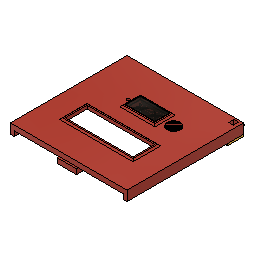
MKTNE_RPI_Shield 3d Files (Autodesk Fusion 360 design; units mm, degrees)
Autodesk Fusion 360 part; units mm, degrees
(part 1 of 2)
sketch "Locking Plug" plane through (0, 0, 0) normal (0, 0, 1) x (1, 0, 0)
  line L0 (0, 0) -> (5.08, 0)
  line L1 (5.08, 0) -> (0, -6.35)
  line L2 (0, 0) -> (0, -6.35) construction
  line L3 (0, -6.35) -> (-10.16, -6.35)
  line L4 (-10.16, -6.35) -> (-10.16, 0)
  line L5 (-10.16, 0) -> (-3.81, 0)
  line L6 (-3.81, 0) -> (-3.81, -1.27)
  line L7 (-3.81, -1.27) -> (-2.54, -1.27)
  line L8 (-2.54, -1.27) -> (-2.54, 0)
  line L9 (-2.54, 0) -> (0, 0)
  dimension "d1" = 5.08
  dimension "d4" = 6.35
  dimension "d5" = 2.54
  dimension "d6" = 1.27
  dimension "d7" = 1.27
  dimension "d60" = 10.16
  constraint coincident L0.start L2.start
  constraint horizontal L0
  constraint perpendicular L0 L2
  constraint parallel L0 L3
  constraint perpendicular L3 L4
  constraint collinear L0 L9
  constraint collinear L5 L9
  constraint parallel L7 L9
  constraint parallel L6 L8
  constraint perpendicular L8 L9
  measures "d1" distance of L0.start L0.end
  measures "d4" distance of L1.end L0.start
  measures "d5" distance of L8.end L0.start
  measures "d6" distance of L6.end L7.end
  measures "d7" distance of L7.end L8.end
  measures "d60" distance of L2 L4
extrude "Extrude1" add sketch "Locking Plug" along normal blind 6.35 makes body 1
hole "Hole1" at (-10.16, -3.175, 3.175) direction (1, 0, 0) diameter 3.81 depth 3.81 tip angle 118 bodies 1
sketch "Wings" plane through (0, 0, 0) normal (0, 1, 0) x (-1, 0, 0)
  line L0 (-5.08, 0) -> (2.54, 0)
  line L1 (2.54, 0) -> (2.54, 6.35)
  line L2 (2.54, 6.35) -> (-5.08, 6.35)
  line L3 (-5.08, 6.35) -> (-5.08, 0)
  line L4 (0, 0) -> (0, 6.35) construction
  line L5 (1.27, 6.35) -> (1.27, 0) construction
  line L6 (1.27, 0) -> (1.27, -1.27)
  line L7 (1.27, -1.27) -> (2.54, -1.27)
  line L8 (2.54, -1.27) -> (2.54, 7.62)
  line L9 (2.54, 7.62) -> (1.27, 7.62)
  line L10 (1.27, 7.62) -> (1.27, 6.35)
  dimension "d14" = 1.27
  dimension "d15" = 1.27
  dimension "d16" = 1.27
  constraint coincident L2 L5.start
  constraint coincident L0 L5.end
  constraint perpendicular L0 L5
  constraint parallel L7 L9
  constraint perpendicular L9 L10
  constraint collinear L6 L10
  constraint parallel L5 L8
  constraint equal L6 L10
  measures "d14" distance of L4 L5
  measures "d15" distance of L8.end L9.end
  measures "d16" distance of L5.start L9.end
extrude "Extrude2" add sketch "Wings" against normal blind 2.54 contours L0 L6 L7 L8 | L2 L8 L9 L10 bodies 1
ref_plane "WorkPlane1" through (1.27, 0.254, 3.175) normal (0, 1, 0) x (-1, 0, 0)
sketch "Top Cover" plane through (0.635, 0.254, 3.175) normal (0, 1, 0) x (1, 0, 0)
  line L0 (-0.635, 3.175) -> (-0.635, -3.175) construction
  line L1 (-0.635, -3.3274) -> (-0.635, -7.1374)
  line L2 (-1.905, -3.3274) -> (-1.905, -4.5974)
  line L3 (-1.905, -4.5974) -> (-8.763, -4.5974)
  line L4 (-8.763, -4.5974) -> (-8.763, -3.3274)
  line L5 (-0.635, -3.3274) -> (-1.905, -3.3274)
  line L6 (-1.905, -4.445) -> (-1.905, -3.175)
  line L7 (-3.175, -4.445) -> (-1.905, -4.445)
  line L8 (-3.175, -2.921) -> (-3.175, 2.921)
  line L9 (-3.175, 2.921) -> (-10.033, 2.921)
  line L10 (-10.033, 2.921) -> (-10.033, -2.921)
  line L11 (-10.033, -2.921) -> (-3.175, -2.921)
  line L12 (-3.175, 4.445) -> (-3.175, -4.445)
  line L13 (-10.795, 3.175) -> (-4.445, 3.175)
  line L14 (-4.445, -3.175) -> (-10.795, -3.175)
  line L15 (4.445, -3.175) -> (-1.905, -3.175) construction
  line L16 (-0.635, 3.3274) -> (-0.635, 145.2626)
  line L17 (-0.635, 3.3274) -> (-1.905, 3.3274)
  line L18 (-1.905, 3.3274) -> (-1.905, 4.5974)
  line L19 (-1.905, 4.5974) -> (-8.763, 4.5974)
  line L20 (-8.763, 4.5974) -> (-8.763, 3.3274)
  line L21 (-1.905, 3.175) -> (4.445, 3.175)
  line L22 (-8.763, 3.3274) -> (-17.653, 3.3274)
  line L23 (-17.653, 3.3274) -> (-17.653, -3.3274)
  line L24 (-17.653, -3.3274) -> (-8.763, -3.3274)
  line L25 (-10.795, 3.175) -> (-10.795, -3.175)
  line L26 (-0.635, -7.1374) -> (-153.035, -7.1374)
  line L27 (-153.035, -7.1374) -> (-153.035, 145.2626)
  line L28 (-153.035, 145.2626) -> (-0.635, 145.2626)
  line L29 (-153.035, 56.3626) -> (-155.575, 56.3626)
  line L30 (-155.575, 56.3626) -> (-155.575, 81.7626)
  line L31 (-155.575, 81.7626) -> (-153.035, 81.7626)
  line L32 (-153.035, 69.0626) -> (-155.575, 69.0626) construction
  line L33 (-0.635, -3.3274) -> (-0.635, 3.3274)
  dimension "d20" = 3.81
  dimension "d22" = 0.1524
  dimension "d23" = 6.858
  dimension "d25" = 0.254
  dimension "d26" = 0.254
  dimension "d27" = 6.858
  dimension "d28" = 0.1524
  dimension "d29" = 0.1524
  dimension "d31" = 152.4
  dimension "d32" = 2.54
  dimension "d33" = 25.4
  dimension "d59" = 6.858
  constraint perpendicular L2 L3
  constraint collinear L2 L6
  constraint perpendicular L3 L4
  constraint perpendicular L8 L9
  constraint perpendicular L9 L10
  constraint perpendicular L8 L11
  constraint parallel L3 L11
  constraint collinear L8 L12
  constraint perpendicular L17 L20
  constraint equal L5 L17
  constraint collinear L2 L18
  constraint perpendicular L17 L18
  constraint collinear L0 L1
  constraint collinear L1 L16
  constraint perpendicular L18 L19
  constraint equal L3 L19
  constraint equal L2 L18
  constraint equal L4 L20
  constraint perpendicular L20 L22
  constraint perpendicular L22 L23
  constraint perpendicular L4 L24
  constraint collinear L17 L22
  constraint perpendicular L26 L27
  constraint perpendicular L16 L28
  constraint perpendicular L1 L26
  constraint equal L26 L27
  constraint coincident L27 L29.start
  constraint coincident L27 L31.end
  constraint midpoint L27 L32.start
  constraint midpoint L30 L32.end
  constraint perpendicular L30 L32
  constraint parallel L29 L31
  constraint perpendicular L29 L30
  constraint perpendicular L27 L32
  measures "d20" distance of L1.start L1.end
  measures "d22" distance of L3 L7
  measures "d23" horizontal distance of L8.start L10.end
  measures "d25" distance of L9 L13
  measures "d26" distance of L11 L14
  measures "d27" distance of L2.end L3.end
  measures "d28" distance of L5 L15
  measures "d29" distance of L17 L21
  measures "d31" distance of L1.end L26.end
  measures "d32" distance of L29.start L29.end
  measures "d33" distance of L29.end L30.end
  measures "d59" distance of L23 L25
extrude "Extrude3" add sketch "Top Cover" along normal blind 6.35 separate body contours L1 L2 L3 L4 L5 L6 L16 L17 L18 L19 L20 L22 L23 L24 L26 L27 L28 | L2 L3 L4 L5 L6 L17 L18 L19 L20 L22 L23 L24 L33 makes body 2
extrude "Extrude4" add sketch "Top Cover" against normal blind 6.604 contours L1 L2 L3 L4 L5 L6 L16 L17 L18 L19 L20 L22 L23 L24 L26 L27 L28 | L27 L29 L30 L31 bodies 2
hole "Hole2" at (-17.018, -3.048, 3.175) direction (-1, 0, 0) diameter 3.81 depth 1.27 tip angle 118 bodies 2
sketch "Hollowing" plane through (0, -6.35, 0) normal (0, -1, 0) x (1, 0, 0)
  line L0 (-1.27, 6.5024) -> (0, 6.5024)
  line L1 (0, 6.5024) -> (0, 10.3124)
  line L2 (0, 10.3124) -> (-152.4, 10.3124)
  line L3 (-152.4, 10.3124) -> (-152.4, -53.1876)
  line L4 (-152.4, -53.1876) -> (-154.94, -53.1876)
  line L5 (-154.94, -53.1876) -> (-154.94, -78.5876)
  line L6 (-154.94, -78.5876) -> (-152.4, -78.5876)
  line L7 (-152.4, -78.5876) -> (-152.4, -142.0876)
  line L8 (-152.4, -142.0876) -> (0, -142.0876)
  line L9 (0, -0.1524) -> (-1.27, -0.1524)
  line L10 (-1.27, -0.1524) -> (-1.27, -1.4224)
  line L11 (-1.27, -1.4224) -> (-8.128, -1.4224)
  line L12 (-8.128, -1.4224) -> (-8.128, -0.1524)
  line L13 (-8.128, -0.1524) -> (-17.018, -0.1524)
  line L14 (-17.018, -0.1524) -> (-17.018, 6.5024)
  line L15 (-17.018, 6.5024) -> (-8.128, 6.5024)
  line L16 (-8.128, 6.5024) -> (-8.128, 7.7724)
  line L17 (-8.128, 7.7724) -> (-1.27, 7.7724)
  line L18 (-1.27, 7.7724) -> (-1.27, 6.5024)
  line L19 (-18.288, 5.08) -> (-18.288, 1.27)
  line L20 (-5.08, -3.9624) -> (-10.668, -3.9624)
  line L21 (-20.828, -2.6924) -> (-20.828, 5.2324)
  line L22 (-20.828, 5.2324) -> (-147.32, 5.2324)
  line L23 (-147.32, 5.2324) -> (-147.32, -137.0076)
  line L24 (-147.32, -137.0076) -> (-5.08, -137.0076)
  line L25 (-5.08, -137.0076) -> (-5.08, -3.9624)
  line L26 (-10.668, -2.6924) -> (-20.828, -2.6924)
  line L27 (-10.668, -2.6924) -> (-10.668, -3.9624)
  line L28 (0, -142.0876) -> (0, -0.1524)
  dimension "d41" = 5.08
  dimension "d42" = 5.08
  dimension "d43" = 2.54
  dimension "d45" = 5.08
  dimension "d46" = 2.54
  dimension "d47" = 2.54
  dimension "d48" = 2.54
  dimension "d128" = 5.588
  constraint perpendicular L20 L21
  constraint perpendicular L21 L22
  constraint perpendicular L24 L25
  constraint perpendicular L23 L24
  constraint perpendicular L22 L23
  constraint perpendicular L21 L26
  constraint perpendicular L20 L27
  measures "d41" distance of L7 L23
  measures "d42" distance of L2 L22
  measures "d43" distance of L19 L21
  measures "d45" distance of L8 L24
  measures "d46" distance of L11 L20
  measures "d47" distance of L13 L26
  measures "d48" distance of L12 L27
  measures "d128" distance of L20.start L20.end
extrude "Extrude5" cut sketch "Hollowing" against normal up to surface (10.414 mm away) contours L20 L21 L22 L23 L24 L25 L26 L27 bodies 2 1
sketch "Back Support Cutaway + Covers" plane through (0, -6.35, 0) normal (0, -1, 0) x (1, 0, 0)
  line L0 (-10.668, -3.9624) -> (-5.08, -3.9624)
  line L1 (-5.08, -3.9624) -> (-5.08, -137.0076)
  line L2 (-147.32, -137.0076) -> (-147.32, 5.2324)
  line L3 (-147.32, 5.2324) -> (-20.828, 5.2324)
  line L4 (-20.828, 5.2324) -> (-20.828, -2.6924)
  line L5 (-20.828, -2.6924) -> (-10.668, -2.6924)
  line L6 (-10.668, -2.6924) -> (-10.668, -3.9624)
  line L7 (-1.27, 6.5024) -> (0, 6.5024)
  line L8 (0, 6.5024) -> (0, 10.3124)
  line L9 (0, 10.3124) -> (-152.4, 10.3124)
  line L10 (-152.4, 10.3124) -> (-152.4, -53.1876)
  line L11 (-152.4, -53.1876) -> (-154.94, -53.1876)
  line L12 (-154.94, -53.1876) -> (-154.94, -78.5876)
  line L13 (-154.94, -78.5876) -> (-152.4, -78.5876)
  line L14 (-152.4, -78.5876) -> (-152.4, -142.0876)
  line L15 (-152.4, -142.0876) -> (0, -142.0876)
  line L16 (0, -142.0876) -> (0, -0.1524)
  line L17 (0, -0.1524) -> (-1.27, -0.1524)
  line L18 (-1.27, -0.1524) -> (-1.27, -1.4224)
  line L19 (-1.27, -1.4224) -> (-8.128, -1.4224)
  line L20 (-8.128, -1.4224) -> (-8.128, -0.1524)
  line L21 (-8.128, -0.1524) -> (-17.018, -0.1524)
  line L22 (-17.018, -0.1524) -> (-17.018, 6.5024)
  line L23 (-17.018, 6.5024) -> (-8.128, 6.5024)
  line L24 (-8.128, 6.5024) -> (-8.128, 7.7724)
  line L25 (-8.128, 7.7724) -> (-1.27, 7.7724)
  line L26 (-1.27, 7.7724) -> (-1.27, 6.5024)
  line L27 (0, -3.9624) -> (-5.08, -3.9624)
  line L28 (-5.08, -137.0076) -> (0, -137.0076)
  line L29 (-147.32, -137.0076) -> (-152.4, -137.0076)
  line L30 (-147.32, 5.2324) -> (-152.4, 5.2324)
  line L31 (-152.4, -53.1876) -> (-147.32, -53.1876)
  line L32 (-152.4, -78.5876) -> (-147.32, -78.5876)
  line L33 (-20.828, 5.2324) -> (-20.828, 10.3124)
  line L34 (0, 6.5024) -> (0, -0.1524)
  line L35 (-17.018, -0.1524) -> (-20.828, -0.1524)
  line L36 (-17.018, -0.1524) -> (-17.018, -2.6924)
  line L37 (-147.32, 5.2324) -> (-147.32, -137.0076)
  constraint coincident L16 L27.start
  constraint perpendicular L1 L27
  constraint coincident L1 L28.start
  constraint coincident L16 L28.end
  constraint coincident L1.end L28.start
  constraint coincident L2.start L29.start
  constraint collinear L28 L29
  constraint coincident L14 L29.end
  constraint coincident L10 L30.end
  constraint perpendicular L10 L30
  constraint coincident L2.end L3.start
  constraint coincident L0.end L1.start
  constraint coincident L10.end L11.start
  constraint coincident L2 L31.end
  constraint perpendicular L2 L31
  constraint coincident L13.end L14.start
  constraint coincident L2 L32.end
  constraint perpendicular L2 L32
  constraint coincident L3.end L4.start
  constraint coincident L9 L33.end
  constraint perpendicular L9 L33
  constraint coincident L7.end L8.start
  constraint coincident L17 L16.end
  constraint coincident L16.end L17.start
  constraint coincident L21.end L22.start
  constraint coincident L4 L35.end
  constraint perpendicular L4 L35
  constraint coincident L5 L36.end
  constraint perpendicular L5 L36
extrude "Extrude7" cut sketch "Back Support Cutaway + Covers" against normal blind 6.35 contours L1 L16 L27 L28 | L2 L14 L29 L32 L37 | L2 L10 L30 L31 L37 bodies 2 1
extrude "Extrude8" add sketch "Back Support Cutaway + Covers" along normal blind 2.54 separate body contours L0 L5 L6 L16 L17 L18 L19 L20 L21 L27 L36 | L7 L17 L18 L19 L20 L21 L22 L23 L24 L25 L26 L34 | L4 L7 L8 L9 L22 L23 L24 L25 L26 L33 L35 makes body 3
sketch "Front Plate Cutouts" plane through (0, 6.604, 0) normal (0, 1, 0) x (-1, 0, 0)
  line L0 (9.398, 0.254) -> (2.54, 0.254)
  line L1 (2.54, 0.254) -> (2.54, 6.096)
  line L2 (2.54, 6.096) -> (9.398, 6.096)
  line L3 (9.398, 6.096) -> (9.398, 0.254)
  line L4 (0, 10.3124) -> (0, -142.0876)
  line L5 (0, -142.0876) -> (152.4, -142.0876)
  line L6 (152.4, -142.0876) -> (152.4, 10.3124)
  line L7 (152.4, 10.3124) -> (0, 10.3124)
  line L8 (84.201, -110.1471) -> (84.201, -21.6281)
  line L9 (84.201, -21.6281) -> (112.649, -21.6281)
  line L10 (112.649, -21.6281) -> (112.649, -110.1471)
  line L11 (112.649, -110.1471) -> (84.201, -110.1471)
  line L12 (39.751, -46.8376) -> (58.801, -46.8376)
  line L13 (58.801, -46.8376) -> (58.801, -84.9376)
  line L14 (58.801, -84.9376) -> (39.751, -84.9376)
  line L15 (84.201, -65.8876) -> (58.801, -65.8876) construction
  line L16 (49.276, -46.8376) -> (49.276, -34.2593) construction
  line L17 (39.751, -65.8876) -> (0, -65.8876) construction
  line L18 (112.649, -65.8876) -> (152.4, -65.8876) construction
  line L19 (84.201, -21.6281) -> (49.276, -21.6281) construction
  line L20 (49.276, -21.6281) -> (49.276, -34.2064) construction
  line L21 (39.751, -84.9376) -> (39.751, -46.8376)
  circle A0 centre (49.276, -91.2876) radius 1.9685
  line L22 (39.751, -84.9376) -> (49.276, -91.2876) construction
  line L23 (49.276, -91.2876) -> (58.801, -84.9376) construction
  line L24 (59.276, -21.6281) -> (59.276, -41.6281)
  line L25 (59.276, -41.6281) -> (39.276, -41.6281)
  line L26 (39.276, -41.6281) -> (39.276, -21.6281)
  line L27 (39.276, -21.6281) -> (59.276, -21.6281)
  line L28 (39.276, -33.7237) -> (47.1804, -41.6281)
  line L29 (39.276, -31.2346) -> (49.6695, -41.6281)
  line L30 (39.276, -34.855) -> (46.0491, -41.6281)
  line L31 (39.276, -41.6281) -> (59.276, -21.6281) construction
  line L32 (39.276, -37.344) -> (43.5601, -41.6281)
  line L33 (39.276, -30.1033) -> (50.8008, -41.6281)
  line L34 (39.276, -27.6143) -> (53.2898, -41.6281)
  line L35 (39.276, -26.4829) -> (54.4212, -41.6281)
  line L36 (39.276, -23.9939) -> (56.9102, -41.6281)
  line L37 (39.276, -22.8625) -> (58.0416, -41.6281)
  line L38 (40.5306, -21.6281) -> (59.276, -40.3735)
  line L39 (39.276, -38.4754) -> (42.4287, -41.6281)
  line L40 (41.662, -21.6281) -> (59.276, -39.2421)
  line L41 (59.276, -36.7531) -> (44.151, -21.6281)
  line L42 (45.2824, -21.6281) -> (59.276, -35.6217)
  line L43 (47.7714, -21.6281) -> (59.276, -33.1327)
  line L44 (48.9028, -21.6281) -> (59.276, -32.0013)
  line L45 (51.3918, -21.6281) -> (59.276, -29.5123)
  line L46 (52.5231, -21.6281) -> (59.276, -28.381)
  line L47 (55.0122, -21.6281) -> (59.276, -25.8919)
  line L48 (56.1435, -21.6281) -> (59.276, -24.7606)
  circle A1 centre (49.276, -31.6281) radius 8.5
  point P0 (40.8523, -40.0518)
  dimension "d61" = 88.519
  dimension "d62" = 28.448
  dimension "d64" = 19.05
  dimension "d65" = 38.1
  dimension "d67" = 25.4
  dimension "d106" = 3.937
  dimension "d107" = 6.35
  dimension "d162" = 20
  dimension "d163" = 20
  dimension "d164" = 0.8
  dimension "d165" = 1.76
  dimension "d166" = 1.76
  dimension "d167" = 0.8
  dimension "d168" = 1.76
  dimension "d169" = 0.8
  dimension "d171" = 1.76
  dimension "d172" = 0.8
  dimension "d173" = 1.76
  dimension "d174" = 0.8
  dimension "d175" = 2.2293
  dimension "d176" = 0.8
  dimension "d177" = 1.76
  dimension "d178" = 0.8
  dimension "d179" = 1.76
  dimension "d180" = 0.8
  dimension "d181" = 1.76
  dimension "d182" = 0.8
  dimension "d183" = 1.76
  dimension "d184" = 0.8
  dimension "d185" = 17
  constraint perpendicular L10 L11
  constraint perpendicular L8 L11
  constraint perpendicular L9 L10
  constraint parallel L6 L10
  constraint parallel L8 L13
  constraint coincident L8 L15.start
  constraint midpoint L13 L15.end
  constraint midpoint L8 L15.start
  constraint perpendicular L13 L15
  constraint midpoint L4 L17.end
  constraint midpoint L10 L18.start
  constraint midpoint L6 L18.end
  constraint collinear L17 L18
  constraint equal L17 L18
  constraint collinear L9 L19
  constraint collinear L16 L20
  constraint equal L16 L20
  constraint perpendicular L14 L21
  constraint perpendicular L12 L21
  constraint perpendicular L12 L13
  constraint coincident L17.start L21
  constraint coincident A0.centre L22.end
  constraint equal L22 L23
  constraint midpoint L12 L16.start
  constraint perpendicular L19 L20
  constraint perpendicular L24 L25
  constraint perpendicular L24 L27
  constraint perpendicular L26 L27
  constraint perpendicular L20 L25
  constraint collinear L19 L27
  constraint midpoint L19.end L27
  constraint coincident L26 L28.start
  constraint coincident L25 L28.end
  constraint coincident L26 L29.start
  constraint coincident L25 L29.end
  constraint parallel L28 L29
  constraint coincident L26 L30.start
  constraint parallel L28 L30
  constraint coincident L25 L30.end
  constraint perpendicular L30 L31
  constraint coincident L26 L32.start
  constraint coincident L25 L32.end
  constraint coincident L26 L33.start
  constraint coincident L25 L33.end
  constraint coincident L26 L34.start
  constraint coincident L25 L34.end
  constraint coincident L26 L35.start
  constraint coincident L25 L35.end
  constraint parallel L34 L35
  constraint parallel L33 L34
  constraint parallel L29 L33
  constraint parallel L30 L32
  constraint coincident L26 L36.start
  constraint coincident L25 L36.end
  constraint coincident L26 L37.start
  constraint coincident L25 L37.end
  constraint parallel L36 L38
  constraint parallel L37 L38
  constraint parallel L35 L36
  constraint coincident L26 L39.start
  constraint coincident L25 L39.end
  constraint parallel L32 L39
  constraint midpoint L39 P0
  constraint coincident L27 L38.start
  constraint coincident L24 L38.end
  constraint coincident L27 L40.start
  constraint coincident L24 L40.end
  constraint coincident L24 L41.start
  constraint coincident L27 L41.end
  constraint parallel L40 L41
  constraint coincident L27 L42.start
  constraint coincident L24 L42.end
  constraint coincident L27 L43.start
  constraint coincident L24 L43.end
  constraint coincident L27 L44.start
  constraint coincident L24 L44.end
  constraint coincident L27 L45.start
  constraint coincident L24 L45.end
  constraint parallel L38 L40
  constraint parallel L41 L42
  constraint parallel L42 L43
  constraint parallel L43 L44
  constraint parallel L44 L45
  constraint coincident L27 L46.start
  constraint coincident L24 L46.end
  constraint coincident L27 L47.start
  constraint coincident L24 L47.end
  constraint coincident L27 L48.start
  constraint coincident L24 L48.end
  constraint parallel L47 L48
  constraint parallel L46 L47
  constraint parallel L45 L46
  constraint midpoint L31 A1.centre
  measures "d61" distance of L9.end L10.end
  measures "d62" distance of L8.end L9.end
  measures "d64" distance of L12.start L12.end
  measures "d65" distance of L14.end L12.start
  measures "d67" distance of L15.start L15.end
  measures "d106" diameter of A0
  measures "d107" distance of L14 A0.centre
  measures "d162" distance of L24.start L24.end
  measures "d163" distance of L24.start L26.end
  measures "d164" distance of L28 L30
  measures "d165" distance of L28 L29
  measures "d166" distance of L30 L32
  measures "d167" distance of L29 L33
  measures "d168" distance of L33 L34
  measures "d169" distance of L34 L35
  measures "d171" distance of L35 L36
  measures "d172" distance of L36 L37
  measures "d173" distance of L37 L38
  measures "d174" distance of L32 L39
  measures "d175" distance of L25.end P0
  measures "d176" distance of L38 L40
  measures "d177" distance of L40 L41
  measures "d178" distance of L41 L42
  measures "d179" distance of L42 L43
  measures "d180" distance of L43 L44
  measures "d181" distance of L44 L45
  measures "d182" distance of L45 L46
  measures "d183" distance of L46 L47
  measures "d184" distance of L47 L48
  measures "d185" diameter of A1
extrude "Extrude11" cut sketch "Front Plate Cutouts" against normal blind 2.54 contours L8 L9 L10 L11 | A0 | L44 A1 | L42 L43 A1 | L40 L41 A1 | L37 L38 A1 | L35 L36 A1 | L33 L34 A1 | L29 A1 bodies 2
sketch "Sketch14" plane through (0, 4.064, 0) normal (0, -1, 0) x (1, 0, 0)
  line L0 (-48.0857, -40.0443) -> (-40.8598, -32.8184)
  line L1 (-55.8809, -36.9784) -> (-43.9257, -25.0232)
  line L2 (-42.6802, -26.2667) -> (-54.6374, -38.2239)
  circle A0 centre (-49.276, -91.2876) radius 1.9685
  line L3 (-57.776, -31.6327) -> (-49.2714, -23.1281)
  line L4 (-47.0729, -23.4186) -> (-57.4855, -33.8312)
  line L5 (-51.4951, -39.8333) -> (-41.0708, -29.409)
  line L6 (-40.776, -31.6033) -> (-49.3008, -40.1281)
  line L7 (-57.2075, -34.6846) -> (-46.2195, -23.6966)
  line L8 (-44.5782, -24.5443) -> (-56.3598, -36.3259)
  line L9 (-112.649, -21.6281) -> (-84.201, -21.6281)
  line L10 (-84.201, -21.6281) -> (-84.201, -110.1471)
  line L11 (-84.201, -110.1471) -> (-112.649, -110.1471)
  line L12 (-112.649, -110.1471) -> (-112.649, -21.6281)
  line L13 (-50.4899, -23.2152) -> (-57.6889, -30.4142)
  line L14 (-53.986, -38.7038) -> (-42.2003, -26.9181)
  line L15 (-41.3502, -28.5571) -> (-52.347, -39.5539)
  line L16 (-20.828, 5.2324) -> (-147.32, 5.2324)
  line L17 (-147.32, 5.2324) -> (-147.32, -137.0076)
  line L18 (-147.32, -137.0076) -> (-5.08, -137.0076)
  line L19 (-5.08, -137.0076) -> (-5.08, -3.9624)
  line L20 (-5.08, -3.9624) -> (-10.668, -3.9624)
  line L21 (-10.668, -3.9624) -> (-10.668, -2.6924)
  line L22 (-10.668, -2.6924) -> (-20.828, -2.6924)
  line L23 (-20.828, -2.6924) -> (-20.828, 5.2324)
  line L24 (-59.276, -21.6281) -> (-59.276, -41.6281)
  line L25 (-59.276, -41.6281) -> (-39.276, -41.6281)
  line L26 (-39.276, -41.6281) -> (-39.276, -21.6281)
  line L27 (-39.276, -21.6281) -> (-59.276, -21.6281)
  arc A1 (-53.986, -38.7038) -> (-52.347, -39.5539) centre (-49.276, -31.6281) ccw
  arc A2 (-41.3502, -28.5571) -> (-42.2003, -26.9181) centre (-49.276, -31.6281) ccw
  arc A3 (-50.4899, -23.2152) -> (-57.6889, -30.4142) centre (-49.276, -31.6281) ccw
  arc A4 (-44.5782, -24.5443) -> (-46.2195, -23.6966) centre (-49.276, -31.6281) ccw
  arc A5 (-57.2075, -34.6846) -> (-56.3598, -36.3259) centre (-49.276, -31.6281) ccw
  arc A6 (-51.4951, -39.8333) -> (-49.3008, -40.1281) centre (-49.276, -31.6281) ccw
  arc A7 (-40.776, -31.6033) -> (-41.0708, -29.409) centre (-49.276, -31.6281) ccw
  arc A8 (-57.776, -31.6327) -> (-57.4855, -33.8312) centre (-49.276, -31.6281) ccw
  arc A9 (-47.0729, -23.4186) -> (-49.2714, -23.1281) centre (-49.276, -31.6281) ccw
  arc A10 (-55.8809, -36.9784) -> (-54.6374, -38.2239) centre (-49.276, -31.6281) ccw
  arc A11 (-42.6802, -26.2667) -> (-43.9257, -25.0232) centre (-49.276, -31.6281) ccw
  arc A12 (-48.0857, -40.0443) -> (-40.8598, -32.8184) centre (-49.276, -31.6281) ccw
  circle A13 centre (-49.276, -31.6281) radius 8.5
  circle A14 centre (-57.276, -23.6281) radius 0.8
  circle A15 centre (-41.276, -23.6281) radius 0.8
  circle A16 centre (-41.276, -39.6281) radius 0.8
  circle A17 centre (-57.276, -39.6281) radius 0.8
  line L28 (-57.276, -39.6281) -> (-41.276, -39.6281) construction
  line L29 (-41.276, -39.6281) -> (-41.276, -23.6281) construction
  line L30 (-41.276, -23.6281) -> (-57.276, -23.6281) construction
  line L31 (-49.276, -39.6281) -> (-49.276, -41.6281) construction
  line L32 (-49.276, -23.6281) -> (-49.276, -21.6281) construction
  dimension "d188" = 16
  dimension "d189" = 1.6
  constraint concentric A1 A13
  constraint coincident L15.start A13
  constraint coincident A17.centre L28.start
  constraint coincident A16.centre L28.end
  constraint coincident A15.centre L29.end
  constraint coincident A14.centre L30.end
  constraint perpendicular L28 L29
  constraint perpendicular L29 L30
  constraint parallel L26 L29
  constraint equal L28 L29
  constraint equal L29 L30
  constraint midpoint L28 L31.start
  constraint midpoint L25 L31.end
  constraint perpendicular L25 L31
  constraint midpoint L30 L32.start
  constraint midpoint L27 L32.end
  constraint equal L31 L32
  constraint equal A15 A16
  constraint equal A16 A17
  constraint equal A14 A17
  measures "d188" distance of A16.centre A15.centre
  measures "d189" diameter of A15
extrude "Extrude21" cut sketch "Sketch14" against normal blind 1.27 contours L0 L6 A13 | L0 A12 A13 | L5 L6 A6 A7 A13 | L5 L15 A13 | L14 L15 A1 A2 A13 | L2 L14 A13 | L1 L2 A10 A11 A13 | L1 L8 A13 | L7 L8 A4 A5 A13 | L4 L7 A13 | L3 L4 A8 A9 A13 | L3 L13 A13 | L13 A3 A13 | A14 | A15 | A16 | A17 bodies 2
extrude "Extrude12" cut sketch "Front Plate Cutouts" against normal blind 1.27 contours L12 L13 L14 L21 bodies 2
sketch "Strike Lights" plane through (0, 5.334, 0) normal (0, 1, 0) x (-1, 0, 0)
  line L0 (39.751, -84.9376) -> (58.801, -84.9376)
  line L1 (58.801, -84.9376) -> (58.801, -46.8376)
  line L2 (58.801, -46.8376) -> (39.751, -46.8376)
  line L3 (39.751, -46.8376) -> (39.751, -84.9376)
  line L4 (39.751, -65.8876) -> (58.801, -65.8876) construction
  line L5 (44.196, -81.2766) -> (44.196, -79.2446)
  line L6 (44.196, -71.5806) -> (44.196, -69.5486)
  line L7 (44.196, -62.2266) -> (44.196, -60.1946)
  line L8 (44.196, -52.5306) -> (44.196, -50.4986)
  line L9 (54.356, -50.4986) -> (54.356, -52.5306)
  line L10 (54.356, -62.2266) -> (54.356, -60.1946)
  line L11 (54.356, -81.2766) -> (54.356, -79.2446)
  line L12 (54.356, -71.5806) -> (54.356, -69.5486)
  line L13 (48.641, -71.6026) -> (49.911, -72.8726)
  line L14 (49.911, -72.8726) -> (49.911, -79.2226)
  line L15 (49.911, -79.2226) -> (48.641, -77.9526)
  line L16 (48.641, -77.9526) -> (48.641, -71.6026)
  line L17 (48.641, -52.5526) -> (49.911, -53.8226)
  line L18 (49.911, -53.8226) -> (49.911, -60.1726)
  line L19 (49.911, -60.1726) -> (48.641, -58.9026)
  line L20 (48.641, -58.9026) -> (48.641, -52.5526)
  line L21 (48.006, -78.0796) -> (48.006, -76.0476)
  line L22 (48.006, -74.7776) -> (48.006, -72.7456)
  line L23 (48.006, -59.0296) -> (48.006, -56.9976)
  line L24 (48.006, -55.7276) -> (48.006, -53.6956)
  line L25 (48.006, -74.7776) -> (44.196, -71.5806)
  line L26 (48.006, -72.7456) -> (44.196, -69.5486)
  line L27 (48.006, -76.0476) -> (44.196, -79.2446)
  line L28 (48.006, -78.0796) -> (44.196, -81.2766)
  line L29 (48.006, -59.0296) -> (44.196, -62.2266)
  line L30 (48.006, -56.9976) -> (44.196, -60.1946)
  line L31 (44.196, -52.5306) -> (48.006, -55.7276)
  line L32 (48.006, -53.6956) -> (44.196, -50.4986)
  line L33 (48.006, -76.0476) -> (48.006, -74.7776) construction
  line L34 (48.641, -77.9526) -> (49.911, -72.8726) construction
  line L35 (48.006, -75.4126) -> (50.546, -75.4126) construction
  line L36 (48.006, -56.9976) -> (48.006, -55.7276) construction
  line L37 (48.641, -58.9026) -> (49.911, -53.8226) construction
  line L38 (48.006, -56.3626) -> (50.546, -56.3626) construction
  line L39 (50.546, -78.0796) -> (50.546, -76.0476)
  line L40 (50.546, -76.0476) -> (50.546, -74.7776) construction
  line L41 (50.546, -74.7776) -> (50.546, -72.7456)
  line L42 (50.546, -74.7776) -> (54.356, -71.5806)
  line L43 (54.356, -69.5486) -> (50.546, -72.7456)
  line L44 (50.546, -76.0476) -> (54.356, -79.2446)
  line L45 (50.546, -78.0796) -> (54.356, -81.2766)
  line L46 (50.546, -59.0296) -> (50.546, -56.9976)
  line L47 (50.546, -56.9976) -> (50.546, -55.7276) construction
  line L48 (50.546, -55.7276) -> (50.546, -53.6956)
  line L49 (50.546, -59.0296) -> (54.356, -62.2266)
  line L50 (54.356, -60.1946) -> (50.546, -56.9976)
  line L51 (50.546, -55.7276) -> (54.356, -52.5306)
  line L52 (50.546, -53.6956) -> (54.356, -50.4986)
  line L53 (49.276, -56.3626) -> (49.276, -46.8376) construction
  line L54 (49.276, -56.3626) -> (49.276, -65.8876) construction
  line L55 (49.276, -65.8876) -> (49.276, -75.4126) construction
  dimension "d111" = 50
  dimension "d112" = 50
  dimension "d113" = 50
  dimension "d114" = 50
  dimension "d115" = 0.635
  dimension "d116" = 2.032
  dimension "d117" = 1.27
  dimension "d118" = 6.35
  dimension "d119" = 1.27
  dimension "d120" = 135
  dimension "d121" = 50
  dimension "d122" = 50
  dimension "d123" = 3.81
  dimension "d124" = 50
  dimension "d125" = 50
  constraint midpoint L3 L4.start
  constraint midpoint L1 L4.end
  constraint collinear L16 L20
  constraint collinear L14 L18
  constraint parallel L13 L15
  constraint parallel L13 L17
  constraint parallel L17 L19
  constraint equal L5 L11
  constraint equal L11 L12
  constraint equal L6 L12
  constraint equal L6 L7
  constraint equal L7 L10
  constraint equal L9 L10
  constraint equal L8 L9
  constraint collinear L5 L6
  constraint collinear L6 L7
  constraint collinear L7 L8
  constraint collinear L9 L10
  constraint collinear L10 L12
  constraint collinear L11 L12
  constraint parallel L10 L18
  constraint parallel L14 L16
  constraint equal L14 L18
  constraint parallel L23 L24
  constraint collinear L21 L22
  constraint collinear L23 L24
  constraint collinear L22 L23
  constraint parallel L8 L20
  constraint perpendicular L4 L18
  constraint parallel L25 L26
  constraint parallel L31 L32
  constraint parallel L27 L28
  constraint parallel L22 L33
  constraint midpoint L34 L35
  constraint midpoint L33 L35.start
  constraint parallel L4 L35
  constraint midpoint L36 L38.start
  constraint midpoint L37 L38
  constraint parallel L35 L38
  constraint parallel L29 L30
  constraint perpendicular L33 L35
  constraint equal L33 L36
  constraint vertical L39
  constraint parallel L39 L40
  constraint parallel L39 L41
  constraint midpoint L35.end L40
  constraint equal L21 L39
  constraint equal L22 L41
  constraint equal L33 L40
  constraint parallel L42 L43
  constraint equal L25 L42
  constraint midpoint L38.end L47
  constraint equal L36 L47
  constraint collinear L47 L48
  constraint collinear L46 L47
  constraint equal L46 L48
  constraint equal L24 L48
  constraint perpendicular L38 L47
  constraint midpoint L37 L53.start
  constraint midpoint L2 L53.end
  constraint midpoint L4 L54.end
  constraint perpendicular L4 L54
  constraint equal L53 L54
  constraint midpoint L34 L55.end
  constraint equal L54 L55
  measures "d111" angle of L6 L26
  measures "d112" angle of L8 L32
  measures "d113" angle of L5 L28
  measures "d114" angle of L7 L29
  measures "d115" distance of L16 L22
  measures "d116" distance of L22.start L22.end
  measures "d117" distance of L21.end L22.start
  measures "d118" distance of L13.end L14.end
  measures "d119" distance of L14 L16
  measures "d120" angle of L14 L15
  measures "d121" angle of L11 L45
  measures "d122" angle of L12 L43
  measures "d123" distance of L6 L22
  measures "d124" angle of L10 L49
  measures "d125" angle of L9 L52
extrude "Extrude13" cut sketch "Strike Lights" against normal blind 1.27 contours L5 L21 L27 L28 | L6 L22 L25 L26 | L7 L23 L29 L30 | L8 L24 L31 L32 | L9 L48 L51 L52 | L10 L46 L49 L50 | L11 L39 L44 L45 | L12 L41 L42 L43 | L13 L14 L15 L16 | L17 L18 L19 L20 bodies 2
sketch "PCB Points + spliter" plane through (0, 4.064, 0) normal (0, -1, 0) x (1, 0, 0)
  line L0 (-44.196, -79.2446) -> (-44.196, -81.2766)
  line L1 (-44.196, -81.2766) -> (-48.006, -78.0796)
  line L2 (-48.006, -78.0796) -> (-48.006, -76.0476)
  line L3 (-48.006, -76.0476) -> (-44.196, -79.2446)
  line L4 (-48.006, -56.9976) -> (-44.196, -60.1946)
  line L5 (-44.196, -60.1946) -> (-44.196, -62.2266)
  line L6 (-44.196, -62.2266) -> (-48.006, -59.0296)
  line L7 (-48.006, -59.0296) -> (-48.006, -56.9976)
  line L8 (-54.356, -62.2266) -> (-54.356, -60.1946)
  line L9 (-54.356, -60.1946) -> (-50.546, -56.9976)
  line L10 (-50.546, -56.9976) -> (-50.546, -59.0296)
  line L11 (-50.546, -59.0296) -> (-54.356, -62.2266)
  line L12 (-48.006, -55.7276) -> (-48.006, -53.6956)
  line L13 (-48.006, -53.6956) -> (-44.196, -50.4986)
  line L14 (-44.196, -50.4986) -> (-44.196, -52.5306)
  line L15 (-44.196, -52.5306) -> (-48.006, -55.7276)
  line L16 (-50.546, -78.0796) -> (-54.356, -81.2766)
  line L17 (-54.356, -81.2766) -> (-54.356, -79.2446)
  line L18 (-54.356, -79.2446) -> (-50.546, -76.0476)
  line L19 (-50.546, -76.0476) -> (-50.546, -78.0796)
  line L20 (-49.911, -79.2226) -> (-49.911, -72.8726)
  line L21 (-49.911, -72.8726) -> (-48.641, -71.6026)
  line L22 (-48.641, -71.6026) -> (-48.641, -77.9526)
  line L23 (-48.641, -77.9526) -> (-49.911, -79.2226)
  line L24 (-49.911, -60.1726) -> (-49.911, -53.8226)
  line L25 (-49.911, -53.8226) -> (-48.641, -52.5526)
  line L26 (-48.641, -52.5526) -> (-48.641, -58.9026)
  line L27 (-48.641, -58.9026) -> (-49.911, -60.1726)
  line L28 (-54.356, -52.5306) -> (-54.356, -50.4986)
  line L29 (-54.356, -50.4986) -> (-50.546, -53.6956)
  line L30 (-50.546, -53.6956) -> (-50.546, -55.7276)
  line L31 (-50.546, -55.7276) -> (-54.356, -52.5306)
  line L32 (-48.006, -72.7456) -> (-44.196, -69.5486)
  line L33 (-44.196, -69.5486) -> (-44.196, -71.5806)
  line L34 (-44.196, -71.5806) -> (-48.006, -74.7776)
  line L35 (-48.006, -74.7776) -> (-48.006, -72.7456)
  line L36 (-54.356, -71.5806) -> (-54.356, -69.5486)
  line L37 (-54.356, -69.5486) -> (-50.546, -72.7456)
  line L38 (-50.546, -72.7456) -> (-50.546, -74.7776)
  line L39 (-50.546, -74.7776) -> (-54.356, -71.5806)
  line L40 (-112.649, -21.6281) -> (-84.201, -21.6281)
  line L41 (-84.201, -21.6281) -> (-84.201, -110.1471)
  line L42 (-84.201, -110.1471) -> (-112.649, -110.1471)
  line L43 (-112.649, -110.1471) -> (-112.649, -21.6281)
  circle A0 centre (-49.276, -91.2876) radius 1.9685
  line L44 (-20.828, 5.2324) -> (-147.32, 5.2324)
  line L45 (-147.32, 5.2324) -> (-147.32, -137.0076)
  line L46 (-147.32, -137.0076) -> (-5.08, -137.0076)
  line L47 (-5.08, -137.0076) -> (-5.08, -3.9624)
  line L48 (-5.08, -3.9624) -> (-10.668, -3.9624)
  line L49 (-10.668, -3.9624) -> (-10.668, -2.6924)
  line L50 (-10.668, -2.6924) -> (-20.828, -2.6924)
  line L51 (-20.828, -2.6924) -> (-20.828, 5.2324)
  circle A1 centre (-98.425, -13.3731) radius 3.175
  circle A2 centre (-98.425, -118.4021) radius 3.175
  circle A3 centre (-17.78, -45.085) radius 3.175
  circle A4 centre (-17.78, -95.885) radius 1.905
  circle A5 centre (-98.425, -118.4021) radius 1.905
  circle A6 centre (-98.425, -13.3731) radius 1.905
  circle A7 centre (-17.78, -45.085) radius 1.905
  circle A8 centre (-17.78, -95.885) radius 3.175
  line L52 (-17.78, -45.085) -> (-17.78, -95.885) construction
  line L53 (-17.78, -70.485) -> (-5.08, -70.485) construction
  line L54 (-98.425, -13.3731) -> (-98.425, -118.4021) construction
  line L55 (-98.425, -65.8876) -> (-147.32, -65.8876) construction
  line L56 (-55.626, -63.9826) -> (-42.926, -63.9826)
  line L57 (-55.626, -67.7926) -> (-42.926, -67.7926)
  line L58 (-55.626, -49.2286) -> (-55.626, -82.5466)
  line L59 (-55.626, -82.5466) -> (-42.926, -82.5466)
  line L60 (-42.926, -82.5466) -> (-42.926, -49.2286)
  line L61 (-42.926, -49.2286) -> (-55.626, -49.2286)
  line L62 (-49.276, -63.9826) -> (-49.276, -67.7926) construction
  line L63 (-42.926, -65.8876) -> (-49.276, -65.8876) construction
  line L64 (-56.896, -47.9586) -> (-41.656, -47.9586)
  line L65 (-41.656, -47.9586) -> (-41.656, -83.8166)
  line L66 (-41.656, -83.8166) -> (-56.896, -83.8166)
  line L67 (-56.896, -83.8166) -> (-56.896, -47.9586)
  line L68 (-42.926, -65.8876) -> (-41.656, -65.8876) construction
  line L69 (-49.276, -49.2286) -> (-49.276, -47.9586) construction
  circle A9 centre (-49.276, -31.6281) radius 8.5
  circle A10 centre (-57.276, -39.6281) radius 0.8
  circle A11 centre (-41.276, -39.6281) radius 0.8
  circle A12 centre (-57.276, -23.6281) radius 0.8
  circle A13 centre (-41.276, -23.6281) radius 0.8
  line L70 (-91.1796, -115.2271) -> (-105.6704, -115.2271) construction
  point P0 (-98.425, -110.1471)
  point P1 (-98.425, -115.2271)
  dimension "d129" = 1.27
  dimension "d130" = 3.81
  dimension "d132" = 50.8
  dimension "d133" = 12.7
  dimension "d136" = 3.81
  dimension "d138" = 1.27
  dimension "d139" = 1.27
  dimension "d140" = 1.27
  dimension "d141" = 1.27
  dimension "d142" = 1.27
  dimension "d143" = 1.27
  dimension "d191" = 5.08
  constraint concentric A1 A6
  constraint concentric A3 A7
  constraint concentric A4 A8
  constraint coincident A2.centre A5.centre
  constraint equal A5 A6
  constraint equal A6 A7
  constraint equal A1 A2
  constraint equal A3 A8
  constraint equal A1 A3
  constraint coincident A3.centre A7.centre
  constraint coincident A4.centre A8.centre
  constraint midpoint L52 L53.start
  constraint midpoint L47 L53.end
  constraint perpendicular L52 L53
  constraint perpendicular L47 L53
  constraint coincident A1.centre A6.centre
  constraint midpoint L54 L55.start
  constraint midpoint L45 L55.end
  constraint perpendicular L45 L55
  constraint perpendicular L54 L55
  constraint equal A4 A7
  constraint perpendicular L58 L59
  constraint perpendicular L59 L60
  constraint perpendicular L58 L61
  constraint parallel L56 L57
  constraint parallel L57 L59
  constraint coincident L56.start L58
  constraint coincident L57.start L58
  constraint coincident L57.end L60
  constraint parallel L17 L58
  constraint midpoint L56 L62.start
  constraint midpoint L57 L62.end
  constraint midpoint L60 L63.start
  constraint midpoint L62 L63.end
  constraint perpendicular L62 L63
  constraint perpendicular L56 L62
  constraint parallel L61 L64
  constraint parallel L59 L66
  constraint parallel L60 L65
  constraint parallel L58 L67
  constraint midpoint L65 L68.end
  constraint collinear L63 L68
  constraint coincident L61 L69.start
  constraint coincident L64 L69.end
  constraint midpoint L61 L69.start
  constraint midpoint L64 L69.end
  constraint perpendicular L61 L69
  constraint coincident L54 P0
  constraint midpoint L42 P0
  constraint perpendicular L54 L70
  constraint tangent A2 L70
  constraint coincident L54 P1
  constraint midpoint L70 P1
  measures "d129" distance of A1 A6
  measures "d130" diameter of A6
  measures "d132" distance of A3.centre A4.centre
  measures "d133" distance of L53.start L53.end
  measures "d136" distance of L56 L57
  measures "d138" distance of L17 L58
  measures "d139" distance of L0 L60
  measures "d140" distance of L0.end L59
  measures "d141" distance of L13.end L61
  measures "d142" distance of L58 L67
  measures "d143" distance of L59 L66
  measures "d191" distance of L42 L70
extrude "Extrude14" add sketch "PCB Points + spliter" along normal blind 5.2578 contours A1 | A2 | A3 | A8 bodies 2
thread "Thread1" "ANSI Metric M Profile 3.0 M3x0.5 6H" major diameter 3.086 minor diameter 2.529 pitch 0.5 angle 60 resizes the face on face at (-15.8774, 0.5588, -45.18) on face at (-99.0317, 2.3114, -15.1789) on face at (-96.6696, 0.5588, -119.1421) on face at (-18.6491, 0.5588, -94.1898) on bodies 2
extrude "Extrude15" add sketch "PCB Points + spliter" along normal blind 2.54 contours L56 L57 L58 L60 | L64 L65 L66 L67 bodies 2
sketch "ArtTop" plane through (0, 6.604, 0) normal (0, 1, 0) x (-1, 0, 0)
  line L0 (58.801, -46.8376) -> (58.801, -84.9376)
  line L1 (58.801, -84.9376) -> (39.751, -84.9376)
  line L2 (39.751, -84.9376) -> (39.751, -46.8376)
  line L3 (39.751, -46.8376) -> (58.801, -46.8376)
  line L4 (84.201, -21.6281) -> (112.649, -21.6281)
  line L5 (112.649, -21.6281) -> (112.649, -110.1471)
  line L6 (112.649, -110.1471) -> (84.201, -110.1471)
  line L7 (84.201, -110.1471) -> (84.201, -21.6281)
  circle A0 centre (49.276, -91.2876) radius 1.9685
  line L8 (9.398, 0.254) -> (2.54, 0.254)
  line L9 (2.54, 0.254) -> (2.54, 6.096)
  line L10 (2.54, 6.096) -> (9.398, 6.096)
  line L11 (9.398, 6.096) -> (9.398, 0.254)
  line L12 (0, 10.3124) -> (0, -142.0876)
  line L13 (0, -142.0876) -> (152.4, -142.0876)
  line L14 (152.4, -142.0876) -> (152.4, 10.3124)
  line L15 (152.4, 10.3124) -> (0, 10.3124)
  line L16 (116.459, -17.8181) -> (116.459, -113.9571)
  line L17 (116.459, -113.9571) -> (80.391, -113.9571)
  line L18 (80.391, -113.9571) -> (80.391, -17.8181)
  line L19 (80.391, -17.8181) -> (116.459, -17.8181)
  line L20 (35.941, -88.7476) -> (35.941, -43.0276)
  line L21 (35.941, -43.0276) -> (62.611, -43.0276)
  line L22 (62.611, -43.0276) -> (62.611, -88.7476)
  line L23 (62.611, -88.7476) -> (35.941, -88.7476)
  arc A1 (52.347, -39.5539) -> (53.986, -38.7038) centre (49.276, -31.6281) ccw
  line L24 (52.347, -39.5539) -> (41.3502, -28.5571)
  arc A2 (42.2003, -26.9181) -> (41.3502, -28.5571) centre (49.276, -31.6281) ccw
  line L25 (42.2003, -26.9181) -> (53.986, -38.7038)
  arc A3 (57.6889, -30.4142) -> (50.4899, -23.2152) centre (49.276, -31.6281) ccw
  line L26 (57.6889, -30.4142) -> (50.4899, -23.2152)
  arc A4 (46.2195, -23.6966) -> (44.5782, -24.5443) centre (49.276, -31.6281) ccw
  line L27 (46.2195, -23.6966) -> (57.2075, -34.6846)
  arc A5 (56.3598, -36.3259) -> (57.2075, -34.6846) centre (49.276, -31.6281) ccw
  line L28 (56.3598, -36.3259) -> (44.5782, -24.5443)
  arc A6 (49.3008, -40.1281) -> (51.4951, -39.8333) centre (49.276, -31.6281) ccw
  line L29 (49.3008, -40.1281) -> (40.776, -31.6033)
  arc A7 (41.0708, -29.409) -> (40.776, -31.6033) centre (49.276, -31.6281) ccw
  line L30 (41.0708, -29.409) -> (51.4951, -39.8333)
  arc A8 (57.4855, -33.8312) -> (57.776, -31.6327) centre (49.276, -31.6281) ccw
  line L31 (57.4855, -33.8312) -> (47.0729, -23.4186)
  arc A9 (49.2714, -23.1281) -> (47.0729, -23.4186) centre (49.276, -31.6281) ccw
  line L32 (49.2714, -23.1281) -> (57.776, -31.6327)
  arc A10 (54.6374, -38.2239) -> (55.8809, -36.9784) centre (49.276, -31.6281) ccw
  line L33 (54.6374, -38.2239) -> (42.6802, -26.2667)
  arc A11 (43.9257, -25.0232) -> (42.6802, -26.2667) centre (49.276, -31.6281) ccw
  line L34 (43.9257, -25.0232) -> (55.8809, -36.9784)
  line L35 (40.8598, -32.8184) -> (48.0857, -40.0443)
  arc A12 (40.8598, -32.8184) -> (48.0857, -40.0443) centre (49.276, -31.6281) ccw
  dimension "d147" = -3.81
  dimension "d148" = -3.81
extrude "Extrude16" add sketch "ArtTop" along normal blind 1.778 contours L16 L17 L18 L19 | L20 L21 L22 L23 bodies 2
chamfer "Chamfer1" distance 2.032 distance2 1.778 8 edges at (-49.276, 8.382, -43.0276) (-35.941, 8.382, -65.8876) (-49.276, 8.382, -88.7476) (-62.611, 8.382, -65.8876) (-80.391, 8.382, -65.8876) (-98.425, 8.382, -17.8181) (-116.459, 8.382, -65.8876) (-98.425, 8.382, -113.9571) measured on face at (-61.341, 8.382, -59.5376) measured on face at (-61.341, 8.382, -59.5376) measured on face at (-61.341, 8.382, -59.5376) measured on face at (-61.341, 8.382, -59.5376) measured on face at (-81.661, 8.382, -80.6408) measured on face at (-81.661, 8.382, -80.6408) measured on face at (-81.661, 8.382, -80.6408) measured on face at (-81.661, 8.382, -80.6408) on bodies 2
sketch "Back Plate Mounting Holes" plane through (0, -6.35, 0) normal (0, 1, 0) x (-1, 0, 0)
  line L0 (20.828, 10.3124) -> (20.828, -0.1524)
  line L1 (20.828, -0.1524) -> (17.018, -0.1524)
  line L2 (17.018, -0.1524) -> (17.018, -2.6924)
  line L3 (17.018, -2.6924) -> (10.668, -2.6924)
  line L4 (10.668, -2.6924) -> (10.668, -3.9624)
  line L5 (10.668, -3.9624) -> (5.08, -3.9624)
  line L6 (5.08, -3.9624) -> (5.08, -137.0076)
  line L7 (5.08, -137.0076) -> (0, -137.0076)
  line L8 (0, -137.0076) -> (0, -142.0876)
  line L9 (0, -142.0876) -> (152.4, -142.0876)
  line L10 (152.4, -142.0876) -> (152.4, -137.0076)
  line L11 (152.4, -137.0076) -> (147.32, -137.0076)
  line L12 (147.32, -137.0076) -> (147.32, 5.2324)
  line L13 (147.32, 5.2324) -> (152.4, 5.2324)
  line L14 (152.4, 5.2324) -> (152.4, 10.3124)
  line L15 (152.4, 10.3124) -> (20.828, 10.3124)
  circle A0 centre (17.78, -95.885) radius 3.175
  circle A1 centre (17.78, -95.885) radius 3.175
  circle A2 centre (17.78, -45.085) radius 3.175
  circle A3 centre (17.78, -45.085) radius 3.175
  circle A4 centre (98.425, -13.3731) radius 3.175
  circle A5 centre (98.425, -13.3731) radius 3.175
  circle A6 centre (98.425, -118.4021) radius 3.175
  circle A7 centre (98.425, -118.4021) radius 3.175
  circle A8 centre (98.425, -118.4021) radius 1.75
  circle A9 centre (98.425, -13.3731) radius 1.75
  circle A10 centre (17.78, -45.085) radius 1.75
  circle A11 centre (17.78, -95.885) radius 1.75
  dimension "d152" = 3.5
  constraint concentric A6 A8
  constraint concentric A4 A9
  constraint concentric A2 A10
  constraint concentric A0 A11
  constraint equal A10 A11
  constraint equal A9 A10
  constraint equal A8 A9
  measures "d152" diameter of A11
sketch "Strike Glass" plane through (0, 5.334, 0) normal (0, 1, 0) x (-1, 0, 0)
  line L0 (44.196, -81.2766) -> (44.196, -79.2446)
  line L1 (44.196, -79.2446) -> (48.006, -76.0476)
  line L2 (48.006, -76.0476) -> (48.006, -78.0796)
  line L3 (48.006, -78.0796) -> (44.196, -81.2766)
  line L4 (44.196, -60.1946) -> (48.006, -56.9976)
  line L5 (48.006, -56.9976) -> (48.006, -59.0296)
  line L6 (48.006, -59.0296) -> (44.196, -62.2266)
  line L7 (44.196, -62.2266) -> (44.196, -60.1946)
  line L8 (54.356, -60.1946) -> (54.356, -62.2266)
  line L9 (54.356, -62.2266) -> (50.546, -59.0296)
  line L10 (50.546, -59.0296) -> (50.546, -56.9976)
  line L11 (50.546, -56.9976) -> (54.356, -60.1946)
  line L12 (48.006, -53.6956) -> (48.006, -55.7276)
  line L13 (48.006, -55.7276) -> (44.196, -52.5306)
  line L14 (44.196, -52.5306) -> (44.196, -50.4986)
  line L15 (44.196, -50.4986) -> (48.006, -53.6956)
  line L16 (54.356, -81.2766) -> (50.546, -78.0796)
  line L17 (50.546, -78.0796) -> (50.546, -76.0476)
  line L18 (50.546, -76.0476) -> (54.356, -79.2446)
  line L19 (54.356, -79.2446) -> (54.356, -81.2766)
  line L20 (49.911, -72.8726) -> (49.911, -79.2226)
  line L21 (49.911, -79.2226) -> (48.641, -77.9526)
  line L22 (48.641, -77.9526) -> (48.641, -71.6026)
  line L23 (48.641, -71.6026) -> (49.911, -72.8726)
  line L24 (49.911, -53.8226) -> (49.911, -60.1726)
  line L25 (49.911, -60.1726) -> (48.641, -58.9026)
  line L26 (48.641, -58.9026) -> (48.641, -52.5526)
  line L27 (48.641, -52.5526) -> (49.911, -53.8226)
  line L28 (54.356, -50.4986) -> (54.356, -52.5306)
  line L29 (54.356, -52.5306) -> (50.546, -55.7276)
  line L30 (50.546, -55.7276) -> (50.546, -53.6956)
  line L31 (50.546, -53.6956) -> (54.356, -50.4986)
  line L32 (44.196, -69.5486) -> (48.006, -72.7456)
  line L33 (48.006, -72.7456) -> (48.006, -74.7776)
  line L34 (48.006, -74.7776) -> (44.196, -71.5806)
  line L35 (44.196, -71.5806) -> (44.196, -69.5486)
  line L36 (54.356, -69.5486) -> (54.356, -71.5806)
  line L37 (54.356, -71.5806) -> (50.546, -74.7776)
  line L38 (50.546, -74.7776) -> (50.546, -72.7456)
  line L39 (50.546, -72.7456) -> (54.356, -69.5486)
  line L40 (39.751, -84.9376) -> (58.801, -84.9376)
  line L41 (58.801, -84.9376) -> (58.801, -46.8376)
  line L42 (58.801, -46.8376) -> (39.751, -46.8376)
  line L43 (39.751, -46.8376) -> (39.751, -84.9376)
  line L44 (39.624, -46.7106) -> (39.624, -85.0646)
  line L45 (39.624, -85.0646) -> (58.928, -85.0646)
  line L46 (58.928, -85.0646) -> (58.928, -46.7106)
  line L47 (58.928, -46.7106) -> (39.624, -46.7106)
  dimension "d157" = 0.127
extrude "Extrude19" add sketch "Strike Glass" along normal blind 3.81 separate body contours L0 L1 L2 L3 | L4 L5 L6 L7 | L8 L9 L10 L11 | L12 L13 L14 L15 | L16 L17 L18 L19 | L20 L21 L22 L23 | L24 L25 L26 L27 | L28 L29 L30 L31 | L32 L33 L34 L35 | L36 L37 L38 L39 | L40 L41 L42 L43 makes body 4
extrude "Extrude20" add 1 faces at (-47.1593, 1.524, -65.2526) along direction (0, -1, 0) blind 2.286 on bodies 2 bodies 2